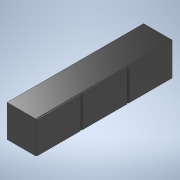
# Autodesk Inventor part: TVBänk
Saved by Autodesk Inventor 2020 (Build 240168000, 168)
## iProperties
Created: 2020-02-25
Part Number: TVBänk
Material: Generic
Document SubType Name: Modeling
Designer: Patrik
Density: 1 g/cm^3
Appearance: Satin - Black
Author: Patrik
Autodesk Inventor part; units mm, degrees
ref_plane "YZ Plane" through (0, 0, 0) normal (1, 0, 0) x (0, 1, 0)
ref_plane "XZ Plane" through (0, 0, 0) normal (0, 1, 0) x (-1, 0, 0)
ref_plane "XY Plane" through (0, 0, 0) normal (0, 0, 1) x (1, 0, 0)
sketch "Sketch1" plane through (0, 0, 0) normal (0, 1, 0) x (-1, 0, 0)
  line L0 (0, 0) -> (380, 0)
  line L1 (380, 0) -> (380, -1800)
  line L2 (380, -1800) -> (0, -1800)
  line L3 (0, -1800) -> (0, 0)
  dimension "d0" = 380
  dimension "d1" = 1800
  constraints: 8 end point, 2 parallel, 1 horizontal, 1 perpendicular
  measures "d0" distance of L1.end L2.end
  measures "d1" distance of L0.end L1.end
extrude "Extrusion1" add sketch "Sketch1" along normal blind 420
sketch "Sketch2" plane through (0, 0, 0) normal (1, 0, 0) x (0, 0, -1)
  line L0 (0, 0) -> (580, 0)
  line L1 (580, 0) -> (580, 420)
  line L2 (580, 420) -> (0, 420)
  line L3 (0, 420) -> (0, 0)
  line L4 (1800, 0) -> (1220, 0)
  line L5 (1220, 0) -> (1220, 420)
  line L6 (1220, 420) -> (1800, 420)
  line L7 (1800, 420) -> (1800, 0)
  line L8 (1800, 420) -> (0, 420) projected
  line L9 (1800, 0) -> (0, 0) projected
  line L10 (600, 420) -> (1200, 420)
  line L11 (1200, 420) -> (1200, 0)
  line L12 (1200, 0) -> (600, 0)
  line L13 (600, 0) -> (600, 420)
  dimension "d4" = 580
  dimension "d6" = 580
  dimension "d7" = 600
  constraints: 24 end point, 6 parallel, 3 horizontal, 3 perpendicular, 2 point on line
  measures "d4" distance of L2.end L1.end
  measures "d6" distance of L5.end L6.end
  measures "d7" distance of L11.end L12.end
extrude "Extrusion2" add sketch "Sketch2" along normal blind 10 contours L3 L2 L1 L0 | L13 L8 L11 L9 | L5 L6 L7 L4
sketch "Sketch3" plane through (0, 420, 0) normal (0, 1, 0) x (1, 0, 0)
  line L0 (-380, 1800) -> (-380, 0) projected
  line L1 (-380, 1800) -> (10, 1800) projected
  line L2 (-380, 0) -> (0, 0)
  line L3 (0, 0) -> (0, 1800)
  line L4 (0, 1800) -> (-380, 1800)
  line L5 (-380, 1800) -> (-380, 0)
  constraints: 8 end point, 2 parallel, 1 horizontal, 1 perpendicular, 1 point on line
extrude "Extrusion3" add sketch "Sketch3" along normal blind 10
sketch "Sketch4" plane through (-380, 0, 0) normal (0, 0, 1) x (1, 0, 0)
  line L0 (0, 0) -> (0, 430) projected
  line L1 (380, 0) -> (380, 420) projected
  line L2 (0, 430) -> (380, 430)
  line L3 (380, 430) -> (380, 0)
  line L4 (380, 0) -> (0, 0)
  line L5 (0, 0) -> (0, 430)
  constraints: 8 end point, 2 parallel, 1 horizontal, 1 perpendicular
extrude "Extrusion4" add sketch "Sketch4" along normal blind 10
sketch "Sketch5" plane through (10, 0, -1800) normal (0, 0, -1) x (-1, 0, 0)
  line L0 (10, 0) -> (10, 430) projected
  line L1 (390, 0) -> (10, 0) projected
  line L2 (10, 430) -> (390, 430)
  line L3 (390, 430) -> (390, 0)
  line L4 (390, 0) -> (10, 0)
  line L5 (10, 0) -> (10, 430)
  constraints: 8 end point, 2 parallel, 1 horizontal, 1 perpendicular
extrude "Extrusion5" add sketch "Sketch5" along normal blind 10
body "Solid1"
